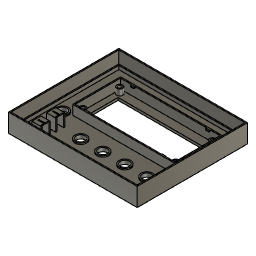
Enclosure_lid2 (Autodesk Fusion 360 design; units mm, degrees)
Autodesk Fusion 360 part; units mm, degrees
sketch "Sketch1" plane through (0, 0, 0) normal (0, 0, 1) x (1, 0, 0)
  line L0 (0, 0) -> (105, 0)
  line L1 (105, 0) -> (105, 90)
  line L2 (105, 90) -> (0, 90)
  line L3 (0, 90) -> (0, 0)
  line L4 (1, 89) -> (104, 89)
  line L5 (104, 89) -> (104, 1)
  line L6 (104, 1) -> (1, 1)
  line L7 (1, 1) -> (1, 89)
  line L8 (2, 88) -> (103, 88)
  line L9 (103, 88) -> (103, 2)
  line L10 (103, 2) -> (2, 2)
  line L11 (2, 2) -> (2, 88)
  dimension "d6" = 105
  dimension "d7" = 90
  dimension "d8" = 88
  dimension "d9" = 103
  dimension "d10" = 1
  dimension "d11" = 1
  dimension "d14" = 86
  dimension "d15" = 101
  dimension "d16" = 1
  dimension "d17" = 1
  constraint horizontal L0
  constraint vertical L1
  constraint horizontal L2
  constraint vertical L3
  constraint coincident L0.start L3.end
  constraint horizontal L4
  constraint vertical L5
  constraint horizontal L6
  constraint vertical L7
  constraint horizontal L8
  constraint vertical L9
  constraint horizontal L10
  constraint vertical L11
  measures "d6" distance of L1.end L2.end
  measures "d7" distance of L0.end L1.end
  measures "d8" distance of L4.end L5.end
  measures "d9" distance of L4.start L4.end
  measures "d10" distance of L2 L4
  measures "d11" distance of L3 L7
  measures "d14" distance of L8.end L9.end
  measures "d15" distance of L8.start L8.end
  measures "d16" distance of L4 L8
  measures "d17" distance of L7 L11
extrude "Extrude1" add sketch "Sketch1" along normal blind 15 contours L0 L1 L2 L3
extrude "Extrude2" add sketch "Sketch1" along normal blind 5 contours L4 L5 L6 L7
extrude "Extrude3" add sketch "Sketch1" along normal blind 2 contours L8 L9 L10 L11
sketch "Sketch2" plane through (0, 0, 2) normal (0, 0, 1) x (-1, 0, 0)
  line L0 (-2, -2) -> (-103, -2)
  line L1 (-103, -2) -> (-103, -88)
  line L2 (-103, -88) -> (-2, -88)
  line L3 (-2, -88) -> (-2, -2)
  line L4 (-21.4, -68) -> (-93.2, -68)
  line L5 (-93.2, -68) -> (-93.2, -43.52)
  line L6 (-93.2, -43.52) -> (-21.4, -43.52)
  line L7 (-21.4, -43.52) -> (-21.4, -68)
  line L8 (-105, 0) -> (-105, -90)
  line L9 (-103, -88) -> (-103, -2)
  line L10 (-2, -88) -> (-103, -88)
  line L11 (-16.48, -74.92) -> (-97.72, -74.92)
  line L12 (-97.72, -74.92) -> (-97.72, -37.92)
  line L13 (-97.72, -37.92) -> (-16.48, -37.92)
  line L14 (-16.48, -37.92) -> (-16.48, -74.92)
  line L15 (-15.48, -75.92) -> (-98.72, -75.92)
  line L16 (-98.72, -75.92) -> (-98.72, -36.92)
  line L17 (-98.72, -36.92) -> (-15.48, -36.92)
  line L18 (-15.48, -36.92) -> (-15.48, -75.92)
  circle A0 centre (-94.92, -71.48) radius 1.45
  circle A1 centre (-94.92, -71.48) radius 2.45
  circle A2 centre (-94.92, -41.36) radius 1.45
  circle A3 centre (-94.92, -41.36) radius 2.45
  circle A4 centre (-19.28, -41.36) radius 1.45
  circle A5 centre (-19.28, -41.36) radius 2.45
  circle A6 centre (-19.28, -71.48) radius 1.45
  circle A7 centre (-19.28, -71.48) radius 2.45
  line L19 (-2, -2) -> (-2, -88)
  dimension "d34" = 24.48
  dimension "d35" = 71.8
  dimension "d39" = 20
  dimension "d40" = 37
  dimension "d41" = 81.24
  dimension "d46" = 4.52
  dimension "d47" = 39
  dimension "d48" = 83.24
  dimension "d49" = 1
  dimension "d51" = 1
  dimension "d55" = 4.9
  dimension "d56" = 2.9
  dimension "d58" = 3.44
  dimension "d59" = 4.9
  dimension "d60" = 2.9
  dimension "d62" = 3.44
  dimension "d63" = 4.9
  dimension "d64" = 2.9
  dimension "d65" = 2.9
  dimension "d66" = 4.9
  dimension "d67" = 3.44
  dimension "d69" = 3.44
  dimension "d76" = 2.8
  dimension "d77" = 2.8
  dimension "d78" = 2.8
  dimension "d79" = 2.8
  dimension "d142" = 19.4
  dimension "d264" = 5.6
  constraint horizontal L4
  constraint vertical L5
  constraint horizontal L6
  constraint vertical L7
  constraint horizontal L11
  constraint vertical L12
  constraint horizontal L13
  constraint vertical L14
  constraint horizontal L15
  constraint vertical L16
  constraint horizontal L17
  constraint vertical L18
  constraint concentric A0 A1
  constraint concentric A2 A3
  constraint concentric A4 A5
  constraint concentric A6 A7
  measures "d34" distance of L4.end L5.end
  measures "d35" distance of L5.end L6.end
  measures "d39" distance of L4 L10
  measures "d40" distance of L11.end L12.end
  measures "d41" distance of L11.start L11.end
  measures "d46" distance of L5 L12
  measures "d47" distance of L15.end L16.end
  measures "d48" distance of L16.end L17.end
  measures "d49" distance of L12 L16
  measures "d51" distance of L13 L17
  measures "d55" diameter of A1
  measures "d56" diameter of A0
  measures "d58" distance of L11 A0.centre
  measures "d59" diameter of A3
  measures "d60" diameter of A2
  measures "d62" distance of L13 A2.centre
  measures "d63" diameter of A7
  measures "d64" diameter of A6
  measures "d65" diameter of A4
  measures "d66" diameter of A5
  measures "d67" distance of L13 A4.centre
  measures "d69" distance of L11 A6.centre
  measures "d76" distance of L14 A6.centre
  measures "d77" distance of L12 A0.centre
  measures "d78" distance of L14 A4.centre
  measures "d79" distance of L12 A2.centre
  measures "d142" distance of L7 L19
  measures "d264" distance of L6 L13
extrude "Extrude4" cut sketch "Sketch2" against normal up to surface (2 mm away) contours L4 L5 L6 L7
extrude "Extrude5" add sketch "Sketch2" along normal blind 4.85 contours A1 | A3 | A5 | A7
extrude "Extrude6" cut sketch "Sketch2" against normal blind 1.2 contours A0 | A2 | A4 | A6
extrude "Extrude7" add sketch "Sketch2" along normal blind 7.75 contours L15 L16 L17 L18
sketch "Sketch4" plane through (0, 74.92, 0) normal (0, -1, 0) x (1, 0, 0)
  line L0 (97.72, 2) -> (97.72, 9.75)
  line L1 (88.72, 9.75) -> (91.72, 9.75)
  line L2 (91.72, 9.75) -> (91.72, 8.75)
  line L3 (91.72, 8.75) -> (88.72, 8.75)
  line L4 (88.72, 8.75) -> (88.72, 9.75)
  line L5 (89.7597, 9.75, 37.796) -> (86.7597, 9.75, 37.796)
  line L6 (86.7597, 9.75, 37.796) -> (86.7597, 8.75, 37.796)
  line L7 (86.7597, 8.75, 37.796) -> (89.7597, 8.75, 37.796)
  line L8 (89.7597, 8.75, 37.796) -> (89.7597, 9.75, 37.796)
  line L9 (97.72, 2, 37) -> (97.72, 9.75, 37)
  line L10 (16.48, 2) -> (97.72, 2)
  line L11 (97.72, 9.75) -> (16.48, 9.75)
  line L12 (97.72, 9.75, 37) -> (16.48, 9.75, 37)
  line L13 (16.48, 9.75) -> (16.48, 2)
  dimension "d103" = 1
  dimension "d104" = 3
  dimension "d105" = 3
  dimension "d106" = 1
  dimension "d108" = 6
  dimension "d109" = 8
  constraint horizontal L1
  constraint vertical L2
  constraint horizontal L3
  constraint vertical L4
  measures "d105" distance of L2.end L3.end
  measures "d106" distance of L1.end L2.end
  measures "d108" distance of L0 L2
extrude "Extrude10" add sketch "Sketch4" against normal blind 1 contours L5 L6 L7 L8 in plane through (0, 37.124, 0) normal (0, -1, 0)
sketch "Sketch5" plane through (0, 0, 2) normal (0, 0, 1) x (-1, 0, 0)
  line L0 (-2, -2) -> (-103, -2)
  line L1 (-103, -2) -> (-103, -88)
  line L2 (-103, -88) -> (-2, -88)
  line L3 (-2, -88) -> (-2, -2)
  line L4 (-15.48, -36.92) -> (-15.48, -75.92)
  line L5 (-15.48, -75.92) -> (-98.72, -75.92)
  line L6 (-98.72, -75.92) -> (-98.72, -36.92)
  line L7 (-98.72, -36.92) -> (-15.48, -36.92)
  circle A0 centre (-36, -22.92) radius 3.6
  circle A1 centre (-54, -22.92) radius 3.6
  circle A2 centre (-72, -22.92) radius 3.6
  circle A3 centre (-90, -22.92) radius 3.6
  circle A4 centre (-36, -22.92) radius 4.75
  circle A5 centre (-54, -22.92) radius 4.75
  circle A6 centre (-72, -22.92) radius 4.75
  circle A7 centre (-90, -22.92) radius 4.75
  line L8 (-103, -88) -> (-103, -2)
  dimension "d116" = 7.2
  dimension "d117" = 7.2
  dimension "d118" = 7.2
  dimension "d119" = 7.2
  dimension "d120" = 9.5
  dimension "d121" = 9.5
  dimension "d122" = 9.5
  dimension "d123" = 9.5
  dimension "d125" = 14
  dimension "d126" = 14
  dimension "d127" = 14
  dimension "d128" = 14
  dimension "d132" = 18
  dimension "d133" = 18
  dimension "d134" = 18
  dimension "d143" = 13
  constraint concentric A0 A4
  constraint concentric A1 A5
  constraint concentric A2 A6
  constraint concentric A3 A7
  measures "d116" diameter of A0
  measures "d117" diameter of A1
  measures "d118" diameter of A2
  measures "d119" diameter of A3
  measures "d120" diameter of A7
  measures "d121" diameter of A6
  measures "d122" diameter of A5
  measures "d123" diameter of A4
  measures "d125" distance of L7 A0.centre
  measures "d126" distance of L7 A1.centre
  measures "d127" distance of L7 A2.centre
  measures "d128" distance of L7 A3.centre
  measures "d132" distance of A0.centre A1.centre
  measures "d133" distance of A1.centre A2.centre
  measures "d134" distance of A2.centre A3.centre
  measures "d143" distance of A3.centre L8
extrude "Extrude11" cut sketch "Sketch5" against normal up to surface (2 mm away) contours A0 | A1 | A2 | A3
extrude "Extrude12" add sketch "Sketch5" along normal blind 1 contours A4 | A5 | A6 | A7
sketch "Sketch6" plane through (0, 0, 2) normal (0, 0, 1) x (-1, 0, 0)
  circle A0 centre (-90, -22.92) radius 4.75
  circle A1 centre (-36, -22.92) radius 4.75
  circle A2 centre (-72, -22.92) radius 4.75
  circle A3 centre (-54, -22.92) radius 4.75
  line L0 (-2, -2) -> (-103, -2)
  line L1 (-103, -2) -> (-103, -88)
  line L2 (-103, -88) -> (-2, -88)
  line L3 (-2, -88) -> (-2, -2)
  line L4 (-15.48, -36.92) -> (-15.48, -75.92)
  line L5 (-15.48, -75.92) -> (-98.72, -75.92)
  line L6 (-98.72, -75.92) -> (-98.72, -36.92)
  line L7 (-98.72, -36.92) -> (-15.48, -36.92)
  circle A4 centre (-16.75, -21.75) radius 1
  circle A5 centre (-16.75, -9.75) radius 1
  line L8 (-14, -19) -> (-19.5, -19)
  line L9 (-19.5, -19) -> (-19.5, -24.5)
  line L10 (-19.5, -24.5) -> (-14, -24.5)
  line L11 (-14, -24.5) -> (-14, -19)
  line L12 (-14, -12.5) -> (-19.5, -12.5)
  line L13 (-19.5, -12.5) -> (-19.5, -7)
  line L14 (-19.5, -7) -> (-14, -7)
  line L15 (-14, -7) -> (-14, -12.5)
  line L16 (-13, -25.5) -> (-20.5, -25.5)
  line L17 (-20.5, -25.5) -> (-20.5, -18)
  line L18 (-20.5, -18) -> (-13, -18)
  line L19 (-13, -18) -> (-13, -25.5)
  line L20 (-13, -13.5) -> (-20.5, -13.5)
  line L21 (-20.5, -13.5) -> (-20.5, -6)
  line L22 (-20.5, -6) -> (-13, -6)
  line L23 (-13, -6) -> (-13, -13.5)
  line L24 (-19.5, -24.5) -> (-20.5, -24.5)
  line L25 (-20.5, -24.5) -> (-20.5, -19)
  line L26 (-20.5, -19) -> (-19.5, -19)
  line L27 (-19.5, -19) -> (-19.5, -24.5)
  line L28 (-19.5, -12.5) -> (-20.5, -12.5)
  line L29 (-20.5, -12.5) -> (-20.5, -7)
  line L30 (-20.5, -7) -> (-19.5, -7)
  line L31 (-19.5, -7) -> (-19.5, -12.5)
  dimension "d146" = 2
  dimension "d147" = 2
  dimension "d148" = 5.5
  dimension "d149" = 5.5
  dimension "d151" = 2.75
  dimension "d152" = 2.75
  dimension "d154" = 12
  dimension "d155" = 5.5
  dimension "d156" = 5.5
  dimension "d157" = 2.75
  dimension "d158" = 2.75
  dimension "d159" = 12
  dimension "d161" = 5
  dimension "d163" = 6.5
  dimension "d165" = 7.5
  dimension "d166" = 7.5
  dimension "d167" = 7.5
  dimension "d168" = 7.5
  dimension "d169" = 1
  dimension "d170" = 1
  dimension "d171" = 1
  dimension "d172" = 1
  dimension "d173" = 5.5
  dimension "d174" = 5.5
  constraint horizontal L8
  constraint vertical L9
  constraint horizontal L10
  constraint vertical L11
  constraint horizontal L12
  constraint vertical L13
  constraint horizontal L14
  constraint vertical L15
  constraint horizontal L16
  constraint vertical L17
  constraint horizontal L18
  constraint vertical L19
  constraint horizontal L20
  constraint vertical L21
  constraint horizontal L22
  constraint vertical L23
  constraint horizontal L24
  constraint vertical L25
  constraint horizontal L26
  constraint vertical L27
  constraint coincident L17 L25.end
  constraint horizontal L28
  constraint vertical L29
  constraint horizontal L30
  constraint vertical L31
  constraint coincident L21 L29.end
  measures "d146" diameter of A5
  measures "d147" diameter of A4
  measures "d148" distance of L8.end L9.end
  measures "d149" distance of L8.start L8.end
  measures "d151" distance of A4.centre L9
  measures "d152" distance of A4.centre L10
  measures "d154" distance of L3 L11
  measures "d155" distance of L12.end L13.end
  measures "d156" distance of L13.end L14.end
  measures "d157" distance of A5.centre L12
  measures "d158" distance of A5.centre L13
  measures "d159" distance of L3 L15
  measures "d161" distance of L0 L14
  measures "d163" distance of L8.end L12.end
  measures "d165" distance of L16.end L17.end
  measures "d166" distance of L17.end L18.end
  measures "d167" distance of L20.end L21.end
  measures "d168" distance of L21.end L22.end
  measures "d169" distance of L14 L22
  measures "d170" distance of L13 L21
  measures "d171" distance of L8 L18
  measures "d172" distance of L9 L17
  measures "d173" distance of L28.end L29.end
  measures "d174" distance of L24.end L25.end
extrude "Extrude13" add sketch "Sketch6" along normal blind 10 contours L8 L10 L11 L16 L17 L18 L19 L24 L26 | L12 L14 L15 L20 L21 L22 L23 L28 L30
extrude "Extrude14" add sketch "Sketch6" along normal blind 1 from surface at 9 contours A4 | A5 | L8 L9 L10 L11 L27 | L12 L13 L14 L15 L31
extrude "Extrude15" cut sketch "Sketch6" against normal up to surface (2 mm away) contours A4 | A5
sketch "Sketch7" plane through (0, 0, 12) normal (0, 0, 1) x (-1, 0, 0)
  line L0 (-20.5, -18) -> (-20.5, -19)
  line L1 (-20.5, -19) -> (-19.5, -19)
  line L2 (-19.5, -19) -> (-19.5, -24.5)
  line L3 (-19.5, -24.5) -> (-20.5, -24.5)
  line L4 (-20.5, -24.5) -> (-20.5, -25.5)
  line L5 (-20.5, -25.5) -> (-13, -25.5)
  line L6 (-13, -25.5) -> (-13, -18)
  line L7 (-13, -18) -> (-20.5, -18)
  line L8 (-14.5, -22.15) -> (-19.5, -22.15)
  line L9 (-19.5, -22.15) -> (-19.5, -21.35)
  line L10 (-19.5, -21.35) -> (-14.5, -21.35)
  line L11 (-14.5, -21.35) -> (-14.5, -22.15)
  line L12 (-14.5, -10.15) -> (-19.5, -10.15)
  line L13 (-19.5, -10.15) -> (-19.5, -9.35)
  line L14 (-19.5, -9.35) -> (-14.5, -9.35)
  line L15 (-14.5, -9.35) -> (-14.5, -10.15)
  line L16 (-13, -13.5) -> (-13, -6)
  line L17 (-19.5, -7) -> (-19.5, -12.5)
  line L18 (-20.5, -13.5) -> (-13, -13.5)
  dimension "d183" = 0.8
  dimension "d184" = 5
  dimension "d185" = 3.35
  dimension "d186" = 0.8
  dimension "d187" = 5
  dimension "d188" = 3.35
  constraint horizontal L8
  constraint vertical L9
  constraint horizontal L10
  constraint vertical L11
  constraint coincident L2 L9.end
  constraint horizontal L12
  constraint vertical L13
  constraint horizontal L14
  constraint vertical L15
  constraint coincident L13 L17.end
  measures "d183" distance of L8.start L10.end
  measures "d184" distance of L9.end L10.end
  measures "d185" distance of L5 L8
  measures "d186" distance of L12.start L14.end
  measures "d187" distance of L13.end L14.end
  measures "d188" distance of L12 L18
extrude "Extrude16" cut sketch "Sketch7" against normal up to surface (1 mm away) contours L2 L8 L9 L10 L11 | L12 L13 L14 L15 L17
sketch "Sketch8" plane through (0, 0, 2) normal (0, 0, 1) x (-1, 0, 0)
  circle A0 centre (-16.75, -9.75) radius 1
  circle A1 centre (-16.75, -21.75) radius 1
  line L0 (-20.5, -6) -> (-13, -6)
  line L1 (-13, -6) -> (-13, -13.5)
  line L2 (-13, -13.5) -> (-20.5, -13.5)
  line L3 (-20.5, -13.5) -> (-20.5, -12.5)
  line L4 (-20.5, -12.5) -> (-14, -12.5)
  line L5 (-14, -12.5) -> (-14, -7)
  line L6 (-14, -7) -> (-20.5, -7)
  line L7 (-20.5, -7) -> (-20.5, -6)
  line L8 (-20.5, -18) -> (-13, -18)
  line L9 (-13, -18) -> (-13, -25.5)
  line L10 (-13, -25.5) -> (-20.5, -25.5)
  line L11 (-20.5, -25.5) -> (-20.5, -24.5)
  line L12 (-20.5, -24.5) -> (-14, -24.5)
  line L13 (-14, -24.5) -> (-14, -19)
  line L14 (-14, -19) -> (-20.5, -19)
  line L15 (-20.5, -19) -> (-20.5, -18)
  circle A2 centre (-90, -22.92) radius 4.75
  circle A3 centre (-36, -22.92) radius 4.75
  circle A4 centre (-72, -22.92) radius 4.75
  circle A5 centre (-54, -22.92) radius 4.75
  line L16 (-2, -2) -> (-103, -2)
  line L17 (-103, -2) -> (-103, -88)
  line L18 (-103, -88) -> (-2, -88)
  line L19 (-2, -88) -> (-2, -2)
  line L20 (-15.48, -36.92) -> (-15.48, -75.92)
  line L21 (-15.48, -75.92) -> (-98.72, -75.92)
  line L22 (-98.72, -75.92) -> (-98.72, -36.92)
  line L23 (-98.72, -36.92) -> (-15.48, -36.92)
  circle A6 centre (-9, -35) radius 3.6
  circle A7 centre (-9, -35) radius 4.75
  dimension "d191" = 7.2
  dimension "d192" = 9.5
  dimension "d194" = 7
  dimension "d196" = 33
  constraint concentric A6 A7
  measures "d191" diameter of A6
  measures "d192" diameter of A7
  measures "d194" distance of L19 A6.centre
  measures "d196" distance of L16 A6.centre
extrude "Extrude17" cut sketch "Sketch8" against normal up to surface (2 mm away) contours A6
extrude "Extrude18" add sketch "Sketch8" along normal blind 1 contours A7
sketch "Sketch15" plane through (0, 0, 0) normal (0, 0, -1) x (1, 0, 0)
  line L0 (0, 0) -> (0, -90)
  line L1 (0, -90) -> (105, -90)
  line L2 (105, -90) -> (105, 0)
  line L3 (105, 0) -> (0, 0)
  line L4 (21.4, -68) -> (21.4, -43.52)
  line L5 (21.4, -43.52) -> (93.2, -43.52)
  line L6 (93.2, -43.52) -> (93.2, -68)
  line L7 (93.2, -68) -> (21.4, -68)
  circle A0 centre (90, -22.92) radius 3.6
  circle A1 centre (36, -22.92) radius 3.6
  circle A2 centre (72, -22.92) radius 3.6
  circle A3 centre (54, -22.92) radius 3.6
  circle A4 centre (16.75, -21.75) radius 1
  circle A5 centre (16.75, -9.75) radius 1
  circle A6 centre (9, -35) radius 3.6
  line L8 (105, -30) -> (0, -30) construction
  dimension "d219" = 30
  constraint coincident L2 L8.start
  constraint coincident L0 L8.end
  constraint perpendicular L0 L8
  measures "d219" distance of L3 L8
sketch "Sketch9" plane through (0, 0, 0) normal (0, 0, -1) x (1, 0, 0)
  circle A0 centre (9, -35) radius 3.6
  circle A1 centre (16.75, -9.75) radius 1
  circle A2 centre (16.75, -21.75) radius 1
  circle A3 centre (54, -22.92) radius 3.6
  circle A4 centre (72, -22.92) radius 3.6
  circle A5 centre (36, -22.92) radius 3.6
  circle A6 centre (90, -22.92) radius 3.6
  line L0 (21.4, -68) -> (21.4, -43.52)
  line L1 (21.4, -43.52) -> (93.2, -43.52)
  line L2 (93.2, -43.52) -> (93.2, -68)
  line L3 (93.2, -68) -> (21.4, -68)
  line L4 (0, 0) -> (0, -90)
  line L5 (0, -90) -> (105, -90)
  line L6 (105, -90) -> (105, 0)
  line L7 (105, 0) -> (0, 0)
  line L8 (95.8964, -30) -> (84.2728, -30) construction
  line L9 (84.2728, -30) -> (84.2728, -35) construction
  line L10 (84.2728, -35) -> (95.8964, -35) construction
  line L11 (95.8964, -35) -> (95.8964, -30) construction
  point P0 (105, -30)
  text T0 "Enter" font "Arial" height 5 align ink ink in box 0 x 0 at (95.8964, -30) x (-1, 0) y (0, -1) spacing 1 height is em
  constraint perpendicular L8 L9
  constraint parallel L8 L10
  constraint parallel L9 L11
  constraint horizontal L8
  constraint coincident L8 P0
extrude "Extrude19" cut sketch "Sketch9" against normal blind 0.4 text T0
sketch "Sketch12" plane through (0, 0, 0) normal (0, 0, -1) x (1, 0, 0)
  line L0 (41.4628, -30) -> (30.7327, -30) construction
  line L1 (30.7327, -30) -> (30.7327, -34.7174) construction
  line L2 (30.7327, -34.7174) -> (41.4628, -34.7174) construction
  line L3 (41.4628, -34.7174) -> (41.4628, -30) construction
  line L4 (17.9199, -48.4505) -> (2.2436, -48.4505) construction
  line L5 (2.2436, -48.4505) -> (2.2436, -53.4505) construction
  line L6 (2.2436, -53.4505) -> (17.9199, -53.4505) construction
  line L7 (17.9199, -53.4505) -> (17.9199, -48.4505) construction
  line L8 (15.9028, -42.6751) -> (3.3796, -42.6751) construction
  line L9 (3.3796, -42.6751) -> (3.3796, -47.6751) construction
  line L10 (3.3796, -47.6751) -> (15.9028, -47.6751) construction
  line L11 (15.9028, -47.6751) -> (15.9028, -42.6751) construction
  line L12 (105, -30) -> (0, -30)
  point P0 (0, -30)
  text T0 "Back" font "Arial" height 4.7174 align ink ink in box 0 x 0 at (41.4628, -30) x (-1, 0) y (0, -1) spacing 1 kerned height is em
  text T1 "Manual" font "Arial" height 5 align ink ink in box 0 x 0 at (17.9199, -48.4505) x (-1, 0) y (0, -1) spacing 1 kerned height is em
  text T2 "Feed" font "Arial" height 5 align ink ink in box 0 x 0 at (15.9028, -42.6751) x (-1, 0) y (0, -1) spacing 1 kerned height is em
  constraint perpendicular L0 L1
  constraint parallel L0 L2
  constraint parallel L1 L3
  constraint perpendicular L4 L5
  constraint parallel L4 L6
  constraint parallel L5 L7
  constraint perpendicular L8 L9
  constraint parallel L8 L10
  constraint parallel L9 L11
  constraint coincident L0 P0
  constraint parallel L0 L12
sketch "Sketch14" plane through (0, 0, 0) normal (0, 0, -1) x (1, 0, 0)
  line L0 (23.4174, -15.9785) -> (9.5625, -15.9785) construction
  line L1 (9.5625, -15.9785) -> (9.5625, -20.9785) construction
  line L2 (9.5625, -20.9785) -> (23.4174, -20.9785) construction
  line L3 (23.4174, -20.9785) -> (23.4174, -15.9785) construction
  line L4 (23.7, -3.6205) -> (8.0139, -3.6205) construction
  line L5 (8.0139, -3.6205) -> (8.0139, -8.6205) construction
  line L6 (8.0139, -8.6205) -> (23.7, -8.6205) construction
  line L7 (23.7, -8.6205) -> (23.7, -3.6205) construction
  text T0 "Power" font "Arial" height 5 align ink ink in box 0 x 0 at (23.4174, -15.9785) x (-1, 0) y (0, -1) spacing 1 kerned height is em
  text T1 "Sensor" font "Arial" height 5 align ink ink in box 0 x 0 at (23.7, -3.6205) x (-1, 0) y (0, -1) spacing 1 kerned height is em
  constraint perpendicular L0 L1
  constraint parallel L0 L2
  constraint parallel L1 L3
  constraint perpendicular L4 L5
  constraint parallel L4 L6
  constraint parallel L5 L7
extrude "Extrude24" cut sketch "Sketch14" against normal blind 0.4 text T1 T0
extrude "Extrude25" add sketch "Sketch2" along normal blind 7.75 contours L15 L16 L17 L18
sketch "Sketch16" plane through (0, 74.92, 0) normal (0, -1, 0) x (1, 0, 0)
  line L0 (16.48, 2) -> (97.72, 2)
  line L1 (97.72, 2) -> (97.72, 9.75)
  line L2 (97.72, 9.75) -> (16.48, 9.75)
  line L3 (25.48, 9.75) -> (28.48, 9.75)
  line L4 (28.48, 9.75) -> (28.48, 8.75)
  line L5 (28.48, 8.75) -> (25.48, 8.75)
  line L6 (25.48, 8.75) -> (25.48, 9.75)
  line L7 (86.72, 9.75) -> (89.72, 9.75)
  line L8 (89.72, 9.75) -> (89.72, 8.75)
  line L9 (89.72, 8.75) -> (86.72, 8.75)
  line L10 (86.72, 8.75) -> (86.72, 9.75)
  line L11 (24.48, 9.75, 37) -> (27.48, 9.75, 37)
  line L12 (27.48, 9.75, 37) -> (27.48, 8.75, 37)
  line L13 (27.48, 8.75, 37) -> (24.48, 8.75, 37)
  line L14 (24.48, 8.75, 37) -> (24.48, 9.75, 37)
  line L15 (89.72, 9.75, 37) -> (86.72, 9.75, 37)
  line L16 (86.72, 9.75, 37) -> (86.72, 8.75, 37)
  line L17 (86.72, 8.75, 37) -> (89.72, 8.75, 37)
  line L18 (89.72, 8.75, 37) -> (89.72, 9.75, 37)
  line L19 (16.48, 2, 37) -> (16.48, 9.75, 37)
  line L20 (97.72, 2, 37) -> (97.72, 9.75, 37)
  line L21 (16.48, 9.75) -> (16.48, 2)
  line L22 (86.7597, 9.75, 37) -> (16.48, 9.75, 37)
  line L23 (97.72, 9.75, 37) -> (89.7597, 9.75, 37)
  dimension "d222" = 3
  dimension "d223" = 1
  dimension "d224" = 3
  dimension "d225" = 1
  dimension "d226" = 3
  dimension "d227" = 1
  dimension "d228" = 3
  dimension "d229" = 1
  dimension "d231" = 8
  dimension "d232" = 8
  dimension "d233" = 8
  constraint horizontal L3
  constraint vertical L4
  constraint horizontal L5
  constraint vertical L6
  constraint coincident L2 L3.start
  constraint horizontal L7
  constraint vertical L8
  constraint horizontal L9
  constraint vertical L10
  constraint coincident L2 L7.start
  measures "d222" distance of L9.end L8.end
  measures "d223" distance of L7.start L9.end
  measures "d226" distance of L4.end L5.end
  measures "d227" distance of L3.end L4.end
  measures "d228" distance of L8.end L9.end
  measures "d229" distance of L7.start L9.end
  measures "d231" distance of L1 L8
extrude "Extrude26" add sketch "Sketch16" along normal blind 1 contours L2 L3 L4 L5 L6 | L2 L7 L8 L9 L10
extrude "Extrude27" add sketch "Sketch16" against normal blind 1 contours L11 L12 L13 L14 L22 | L15 L16 L17 L18 L22 in plane through (0, 37.92, 0) normal (0, -1, 0)
chamfer "Chamfer2" distance 0.6 angle 45 4 edges at (25.98, 38.92, 9.75) (88.22, 38.92, 9.75) (88.22, 73.92, 9.75) (26.98, 73.92, 9.75)
sketch "Sketch17" plane through (0, 0, 0) normal (0, 0, -1) x (1, 0, 0)
  line L0 (72, -34.763) -> (73.9, -31.4721)
  line L1 (72, -34.763) -> (75.6074, -34.763) construction
  line L2 (72, -34.763) -> (70.1, -31.4721)
  line L3 (72, -34.763) -> (75.8739, -34.763) construction
  line L4 (71, -30) -> (73, -30)
  line L5 (71, -30) -> (71, -31.4721)
  line L6 (73, -30) -> (73, -31.4721)
  line L7 (73.9, -31.4721) -> (73, -31.4721)
  line L8 (71, -31.4721) -> (70.1, -31.4721)
  line L9 (105, -90) -> (105, 0)
  point P0 (84.2728, -30)
  dimension "d239" = 60
  dimension "d240" = 120
  dimension "d244" = 3.8
  dimension "d245" = 3.8
  dimension "d247" = 2
  dimension "d249" = 0.9
  dimension "d252" = 32
  constraint horizontal L1
  constraint horizontal L3
  constraint horizontal L4
  constraint coincident L5.end L7
  constraint perpendicular L5 L7
  constraint perpendicular L4 L6
  constraint coincident L4 P0
  constraint collinear L7 L8
  measures "d239" angle of L0 L1
  measures "d240" angle of L2 L3
  measures "d244" distance of L0.start L0.end
  measures "d245" distance of L0.start L2.end
  measures "d247" distance of L4.start L4.end
  measures "d249" distance of L0.end L6
  measures "d252" distance of L6 L9
extrude "Extrude28" cut sketch "Sketch17" against normal blind 0.4
sketch "Sketch18" plane through (0, 0, 0) normal (0, 0, -1) x (1, 0, 0)
  line L0 (71, -30) -> (47.7059, -30) construction
  line L1 (72, -34.763) -> (47.5833, -34.763) construction
  line L2 (53.9986, -30) -> (55.8986, -33.2909)
  line L3 (53.9986, -30) -> (55.9849, -30) construction
  line L4 (53.9986, -30) -> (52.0986, -33.2909)
  line L5 (52.9986, -34.763) -> (54.9986, -34.763)
  line L6 (52.9986, -34.763) -> (52.9986, -33.2909)
  line L7 (54.9986, -34.763) -> (54.9986, -33.2909)
  line L8 (52.0986, -33.2909) -> (52.9986, -33.2909)
  line L9 (54.9986, -33.2909) -> (55.8986, -33.2909)
  point P0 (71, -30)
  point P1 (72, -34.763)
  dimension "d253" = 60
  dimension "d254" = 3.8
  dimension "d255" = 3.8
  dimension "d256" = 60
  dimension "d257" = 2
  dimension "d258" = 0.9
  constraint coincident P0 L0.start
  constraint horizontal L0
  constraint coincident P1 L1.start
  constraint horizontal L1
  constraint horizontal L3
  constraint coincident L0 L2.start
  constraint coincident L1 L5.start
  constraint parallel L1 L5
  constraint perpendicular L6 L8
  constraint coincident L7.end L8
  constraint perpendicular L7 L8
  constraint collinear L8 L9
  measures "d253" angle of L2 L3
  measures "d254" distance of L2.start L2.end
  measures "d255" distance of L2.start L4.end
  measures "d256" angle of L2 L4
  measures "d257" distance of L5.start L5.end
  measures "d258" distance of L4.end L6
extrude "Extrude29" cut sketch "Sketch18" against normal blind 0.4
extrude "Extrude30" cut sketch "Sketch12" against normal blind 0.4 text T1 T2 T0
equation "Outter_wall_width = 105 mm"
equation "Outter_wall_length = 90 mm"
equation "Middle_wall_width = 103 mm"
equation "Middle_wall_lenght = 88 mm"
equation "Side_wall_width = 1 mm"
equation "d6 = Outter_wall_width"
equation "d7 = Outter_wall_length"
equation "d8 = Middle_wall_lenght"
equation "d9 = Middle_wall_width"
equation "d10 = Side_wall_width"
equation "d11 = Side_wall_width"
equation "Inner_wall_width = 101 mm"
equation "Inner_wal_length = 86 mm"
equation "d14 = Inner_wal_length"
equation "d15 = Inner_wall_width"
equation "d16 = Side_wall_width"
equation "d17 = Side_wall_width"
equation "Top_thickness = 2 mm"
equation "Screen_width = 71.8 mm"
equation "Screen_length = 24.48 mm"
equation "Side_t_screen = 19.4 mm"
equation "Top_to_screen = 20 mm"
equation "Screen_pcb_width = 81.24 mm"
equation "Screen_pcb_length = 37 mm"
equation "button_diameter = 7.2 mm"
equation "Inner_wall_height = 5 mm"
equation "Outter_wall_height = 15 mm"
equation "d28 = Outter_wall_height"
equation "d30 = Inner_wall_height"
equation "d32 = Top_thickness"
equation "d34 = Screen_length"
equation "d35 = Screen_width"
equation "d39 = Top_to_screen"
equation "d40 = Screen_pcb_length"
equation "d41 = Screen_pcb_width"
equation "Top_pcb_to_screen = 5.6 mm"
equation "Bottom_pcb_to_screen = 6.95 mm"
equation "Right_pcb_to_screen = 4.52 mm"
equation "d46 = Right_pcb_to_screen"
equation "d47 = Screen_pcb_length + 2 mm"
equation "d48 = Screen_pcb_width + 2 mm"
equation "d49 = Holder_wall_width"
equation "Holder_wall_width = 1 mm"
equation "d51 = Holder_wall_width"
equation "Screen_mount_hole_dia = 2.9 mm"
equation "Screen_mount_outter_hole_dia = 4.9 mm"
equation "Screen_mount_hole_top_edge_distance = 3.44 mm"
equation "d55 = Screen_mount_outter_hole_dia"
equation "d56 = Screen_mount_hole_dia"
equation "d58 = Screen_mount_hole_top_edge_distance"
equation "d59 = Screen_mount_outter_hole_dia"
equation "d60 = Screen_mount_hole_dia"
equation "d62 = Screen_mount_hole_top_edge_distance"
equation "d63 = Screen_mount_outter_hole_dia"
equation "d64 = Screen_mount_hole_dia"
equation "d65 = Screen_mount_hole_dia"
equation "d66 = Screen_mount_outter_hole_dia"
equation "d67 = Screen_mount_hole_top_edge_distance"
equation "d69 = Screen_mount_hole_top_edge_distance"
equation "Screen_mount_hole_side_edge_distance = 2.8 mm"
equation "d76 = Screen_mount_hole_side_edge_distance"
equation "d77 = Screen_mount_hole_side_edge_distance"
equation "d78 = Screen_mount_hole_side_edge_distance"
equation "d79 = Screen_mount_hole_side_edge_distance"
equation "Mount_gol_height = 4.85 mm"
equation "d81 = Mount_gol_height"
equation "Screen_pcb_thickness = 1.9 mm"
equation "Holder_wallheight = 5.85 mm + Screen_pcb_thickness"
equation "d87 = Holder_wallheight"
equation "Lip_width = 2 mm"
equation "Lip_lenght = 1 mm"
equation "Lip_height = 1 mm"
equation "Lip_bottom_distance = 6 mm"
equation "Lip_width2 = 3 mm"
equation "d103 = Lip_lenght"
equation "d104 = Lip_width2"
equation "d105 = Lip_width2"
equation "d106 = Lip_lenght"
equation "Lip_distance_from_right = 8 mm"
equation "d108 = Lip_bottom_distance"
equation "d109 = Lip_distance_from_right"
equation "d112 = -Lip_height"
equation "Button_outter_dia = 9.5 mm"
equation "d116 = button_diameter"
equation "d117 = button_diameter"
equation "d118 = button_diameter"
equation "d119 = button_diameter"
equation "d120 = Button_outter_dia"
equation "d121 = Button_outter_dia"
equation "d122 = Button_outter_dia"
equation "d123 = Button_outter_dia"
equation "Button_hole_to_screen = 14 mm"
equation "d125 = Button_hole_to_screen"
equation "d126 = Button_hole_to_screen"
equation "d127 = Button_hole_to_screen"
equation "d128 = Button_hole_to_screen"
equation "Firs_button_distance = 13 mm"
equation "Button_spacing = 18 mm"
equation "d132 = Button_spacing"
equation "d133 = Button_spacing"
equation "d134 = Button_spacing"
equation "Button_lift = 1 mm"
equation "d138 = Button_lift"
equation "LED_dia = 2 mm"
equation "LED_height = 10 mm"
equation "d142 = Side_t_screen"
equation "d143 = Firs_button_distance"
equation "Led_width = 5.5 mm"
equation "Led_slit_width = 5 mm"
equation "d146 = LED_dia"
equation "d147 = LED_dia"
equation "d148 = Led_width"
equation "d149 = Led_width"
equation "led_hole_to_edge = 2.75 mm"
equation "d151 = led_hole_to_edge"
equation "d152 = led_hole_to_edge"
equation "Led_holder_to_edge = 12 mm"
equation "d154 = Led_holder_to_edge"
equation "d155 = Led_width"
equation "d156 = Led_width"
equation "d157 = led_hole_to_edge"
equation "d158 = led_hole_to_edge"
equation "d159 = Led_holder_to_edge"
equation "first_led_to_bottom = 5 mm"
equation "d161 = first_led_to_bottom"
equation "first_led_to_second = 6.5 mm"
equation "d163 = first_led_to_second"
equation "led_outter_wall_width = Led_width + 2 mm"
equation "d165 = led_outter_wall_width"
equation "d166 = led_outter_wall_width"
equation "d167 = led_outter_wall_width"
equation "d168 = led_outter_wall_width"
equation "d173 = Led_width"
equation "d174 = Led_width"
equation "d175 = LED_height"
equation "d177 = LED_height - 1 mm"
equation "led_slit_length = 0.8 mm"
equation "d183 = led_slit_length"
equation "d184 = Led_slit_width"
equation "d186 = led_slit_length"
equation "d187 = Led_slit_width"
equation "d191 = button_diameter"
equation "d192 = Button_outter_dia"
equation "manual_button_to_edge = 7 mm"
equation "d194 = manual_button_to_edge"
equation "manual_to_bottom = 33 mm"
equation "d196 = manual_to_bottom"
equation "d199 = Button_lift"
equation "distance_letters_to_screen = 14.6 mm"
equation "d220 = Holder_wallheight"
equation "d222 = Lip_width2"
equation "d223 = Lip_lenght"
equation "d224 = Lip_width2"
equation "d225 = Lip_lenght"
equation "d226 = Lip_width2"
equation "d227 = Lip_lenght"
equation "d228 = Lip_width2"
equation "d229 = Lip_lenght"
equation "d231 = Lip_distance_from_right"
equation "d232 = Lip_distance_from_right"
equation "d233 = Lip_distance_from_right"
equation "d234 = Lip_height"
equation "d236 = -Lip_height"
equation "Triangl_side_length = 3.8 mm"
equation "d244 = Triangl_side_length"
equation "d245 = Triangl_side_length"
equation "bottom_triangle_width = 2 mm"
equation "d247 = bottom_triangle_width"
equation "triangle_bottom_to_edge = 0.9 mm"
equation "d249 = triangle_bottom_to_edge"
equation "d254 = Triangl_side_length"
equation "d255 = Triangl_side_length"
equation "d257 = bottom_triangle_width"
equation "d258 = triangle_bottom_to_edge"
equation "d264 = Top_pcb_to_screen"
